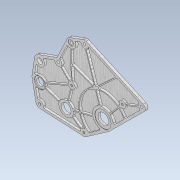
# Autodesk Inventor part: 脚フレーム内側後改
Saved by Autodesk Inventor 2020.2 (Build 242310000, 310)
## iProperties
Created: 2020-02-04
Part Number: 脚フレーム内側後改
Material: アルミニウム 7075
Document SubType Name: Modeling
Designer: aoyam
Density: 2.81 g/cm^3
Appearance: サテン - ブラシ仕上げ 重厚
Mass: 23.6517 g
Surface Area: 186.096 cm^2
Volume: 8.41698 cm^3
Author: aoyam
Autodesk Inventor part; units mm, degrees
ref_plane "YZ Plane" through (0, 0, 0) normal (1, 0, 0) x (0, 1, 0)
ref_plane "XZ Plane" through (0, 0, 0) normal (0, 1, 0) x (-1, 0, 0)
ref_plane "XY Plane" through (0, 0, 0) normal (0, 0, 1) x (1, 0, 0)
sketch "スケッチ2" plane through (0, 0, 0) normal (0, 0, 1) x (1, 0, 0)
  line L0 (0, 0) -> (0, 13.1)
  line L1 (26.2, 7.30753) -> (26.2, 0)
  line L2 (-139.706094, -70) -> (112.711025, -70)
  line L3 (-139.706094, -20) -> (112.711025, -20)
  line L4 (-139.723118, -25) -> (112.694001, -25)
  circle A0 centre (0, 0) radius 20.05
  circle A1 centre (14.844729, 16.628971) radius 2.05
  circle A2 centre (14.844729, 16.628971) radius 14
  circle A3 centre (19.387849, -11) radius 2.05
  circle A4 centre (19.387849, -11) radius 14
  circle A5 centre (0, 0) radius 9.1
  line L5 (0, 0) -> (-93.6, 0)
  circle A6 centre (-93.6, 0) radius 25.1
  circle A7 centre (-52.665625, 10.257531) radius 17.1
  circle A8 centre (-23.2, 0) radius 14.1
  line L6 (0, 0) -> (93.6, 0)
  circle A9 centre (93.6, 0) radius 25.1
  circle A10 centre (52.665625, 10.257531) radius 17.1
  circle A11 centre (23.2, 0) radius 14.1
  dimension "d137" = 7.30753
  dimension "d142" = 70
  dimension "d143" = 50
  dimension "d145" = 45
  dimension "d153" = 4.1
  dimension "d154" = 28
  dimension "d155" = 4.1
  dimension "d156" = 28
  dimension "d157" = 22.291
  dimension "d158" = 22.291
  dimension "d159" = 40.1
  dimension "d160" = 18.2
  dimension "d161" = 93.6
  dimension "d162" = 50.2
  dimension "d164" = 34.2
  dimension "d165" = 28.2
  constraints: 14 end point, 12 centre point, 7 coincident, 5 tangent, 4 symmetric about line, 2 horizontal, 2 parallel, 2 point on line, 1 vertical, 3 other
  measures "d137" distance of L1.start L1.end
  measures "d142" distance from line of L2 point (0, 0)
  measures "d143" distance between parallel lines of L2 L3
  measures "d145" distance between parallel lines of L2 L4
  measures "d153" diameter of A1
  measures "d154" diameter of A2
  measures "d155" diameter of A3
  measures "d156" diameter of A4
  measures "d157" distance of A1.centre point (0, 0)
  measures "d158" distance of A3.centre point (0, 0)
  measures "d159" diameter of A0
  measures "d160" diameter of A5
  measures "d161" distance of L0.start L5.end
  measures "d162" diameter of A6
  measures "d164" diameter of A7
  measures "d165" diameter of A8
sketch "スケッチ6" plane through (0, 0, 0) normal (0, 0, 1) x (1, 0, 0)
  circle A0 centre (93.6, 0) radius 6.025
  circle A1 centre (93.788626, 0) radius 8.025
  circle A2 centre (23.2, 0) radius 4
  circle A3 centre (23.2, 0) radius 14.1 construction
  circle A4 centre (93.6, 0) radius 25.1 construction
  circle A5 centre (23.2, 0) radius 16 construction
  circle A6 centre (93.6, 0) radius 27 construction
  line L0 (93.6, 0) -> (43.961305, 30) construction
  line L1 (43.961305, 30) -> (43.961305, 0) construction
  line L2 (93.6, 0) -> (0, 0)
  circle A7 centre (43.961305, 30) radius 1.5
  circle A8 centre (52.665625, -10.257531) radius 5.5
  circle A9 centre (52.665625, -10.257531) radius 17.1 construction
  circle A10 centre (52.665625, -10.257531) radius 19 construction
  line L3 (10.458367, 21.878509) -> (52.665625, 69.111596)
  line L4 (10.458367, -13.121491) -> (10.458367, 21.878509)
  line L5 (25.458367, -28.121491) -> (10.458367, -13.121491)
  line L6 (95.208425, -28.121491) -> (25.458367, -28.121491)
  line L7 (52.665625, 69.111596) -> (73.258556, 65.895552)
  line L8 (73.258556, 65.895552) -> (144.272455, 39.050636)
  line L9 (144.272455, 39.050636) -> (95.208425, -28.121491)
  circle A11 centre (73.258556, 61.870258) radius 1.5
  circle A12 centre (136.685646, 33.221118) radius 1.5
  line L10 (24.034996, -23.055024) -> (45.351309, -15.50165)
  arc A13 (45.351309, -15.50165) -> (58.061671, -17.460495) centre (52.665625, -10.257531) ccw
  line L11 (58.061671, -17.460495) -> (71.015612, -25.49562)
  arc A14 (71.015612, -25.49562) -> (74.255733, -25.093314) centre (72.402373, -23.4155) ccw
  line L12 (74.255733, -25.093314) -> (88.955218, -8.855845)
  arc A15 (88.955218, -8.855845) -> (101.830891, 5.679122) centre (93.6, 0) ccw
  line L13 (101.830891, 5.679122) -> (117.034634, 23.219838)
  arc A16 (117.034634, 23.219838) -> (113.256379, 26.49471) centre (115.145507, 24.857274) ccw
  line L14 (113.256379, 26.49471) -> (98.052637, 8.953995)
  arc A17 (98.052637, 8.953995) -> (85.704965, 6.13746) centre (93.6, 0) ccw
  line L15 (85.704965, 6.13746) -> (59.901593, 17.294675)
  arc A18 (59.901593, 17.294675) -> (59.314048, 17.467033) centre (58.90939, 15) ccw
  line L16 (59.314048, 17.467033) -> (23.604658, 23.324307)
  arc A19 (23.604658, 23.324307) -> (20.7, 20.857274) centre (23.2, 20.857274) ccw
  line L17 (20.7, 20.857274) -> (20.7, 5.454356)
  arc A20 (20.7, 5.454356) -> (20.7, -5.454356) centre (23.2, 0) ccw
  line L18 (20.7, -5.454356) -> (20.7, -20.69859)
  arc A21 (20.7, -20.69859) -> (24.034996, -23.055024) centre (23.2, -20.69859) ccw
  line L19 (25.7, 5.454356) -> (25.7, 17.913801)
  line L20 (25.7, 17.913801) -> (55.832623, 12.971263)
  line L21 (55.832623, 12.971263) -> (51.789591, -1.300268)
  arc A22 (51.789591, -1.300268) -> (43.681318, -10.788782) centre (52.665625, -10.257531) ccw
  line L22 (43.681318, -10.788782) -> (25.7, -17.16041)
  line L23 (25.7, -17.16041) -> (25.7, -5.454356)
  arc A23 (25.7, -5.454356) -> (25.7, 5.454356) centre (23.2, 0) ccw
  circle A24 centre (58.90939, 15) radius 1.5
  circle A25 centre (72.402373, -23.4155) radius 1.5
  circle A26 centre (23.2, 20.857274) radius 3
  circle A27 centre (115.145507, 24.857274) radius 1.5
  circle A28 centre (23.2, -20.69859) radius 1.5
  circle A29 centre (23.2, 0) radius 5
  circle A30 centre (93.6, 0) radius 5.525 construction
  line L24 (57.614258, -2.740149) -> (61.452441, 12.786227)
  line L25 (61.452441, 12.786227) -> (84.545331, 2.801007)
  arc A31 (84.545331, 2.801007) -> (85.779798, -5.785259) centre (94.081299, -0.209859) ccw
  line L26 (85.779798, -5.785259) -> (73.014253, -20.85157)
  line L27 (73.014253, -20.85157) -> (61.080634, -13.449335)
  arc A32 (61.080634, -13.449335) -> (57.614258, -2.740149) centre (52.665625, -10.257531) ccw
  circle A33 centre (52.665625, -10.257531) radius 4
  line L28 (6.354093, -32.225765) -> (150, -32.225765)
  line L29 (150, -32.225765) -> (150, 70)
  line L30 (150, 70) -> (6.354093, 70)
  line L31 (6.354093, 70) -> (6.354093, -32.225765)
  point P0 (52.665625, 10.257531)
  dimension "d166" = 12.05
  dimension "d167" = 16.05
  dimension "d169" = 8
  dimension "d170" = 28.2
  dimension "d172" = 50.2
  dimension "d173" = 32
  dimension "d175" = 54
  dimension "d176" = 58
  dimension "d177" = 30
  dimension "d178" = 3
  dimension "d191" = 34.2
  dimension "d220" = 6
  dimension "d456" = 2.5
  dimension "d457" = 3
  dimension "d458" = 2.5
  dimension "d459" = 3
  dimension "d460" = 3
  dimension "d461" = 2.5
  dimension "d462" = 2.5
  dimension "d463" = 1
  dimension "d464" = 5
  dimension "d465" = 5
  dimension "d466" = 5
  dimension "d467" = 5
  dimension "d468" = 11
  dimension "d469" = 3.5
  dimension "d470" = 3.5
  dimension "d471" = 3.5
  dimension "d472" = 2
  dimension "d473" = 2
  constraints: 64 end point, 32 centre point, 26 point on circle, 13 concentric, 5 coincident, 3 horizontal, 3 vertical, 2 parallel, 2 tangent, 1 perpendicular, 1 point on line, 5 other
  measures "d166" diameter of A0
  measures "d167" diameter of A1
  measures "d169" diameter of A2
  measures "d170" diameter of A3
  measures "d172" diameter of A4
  measures "d173" diameter of A5
  measures "d175" diameter of A6
  measures "d176" distance of L0.start L0.end
  measures "d177" distance of L0.end L1.end
  measures "d178" diameter of A7
  measures "d191" diameter of A9
  measures "d220" diameter of A26
  measures "d456" radius of A19
  measures "d457" diameter of A28
  measures "d458" radius of A21
  measures "d459" diameter of A24
  measures "d460" diameter of A25
  measures "d461" radius of A14
  measures "d462" radius of A16
  measures "d463" radial gap between concentric circles of A27 A16
  measures "d464" distance between parallel lines of L19 L17
  measures "d465" distance between parallel lines of L23 L18
  measures "d466" distance between parallel lines of L10 L22
  measures "d467" distance between parallel lines of L27 L11
  measures "d468" diameter of A8
  measures "d469" radial gap between concentric circles of A8 A22
  measures "d470" radial gap between concentric circles of A32 A8
  measures "d471" radial gap between concentric circles of A13 A8
  measures "d472" radial gap between concentric circles of A2 A20
  measures "d473" radial gap between concentric circles of A23 A2
extrude "押し出し4" add sketch "スケッチ6" along normal blind 3 contours A1 | L2 A29 A2 | A2 L2 A29 | A31 L26 L27 A32 L24 L2 | L2 L24 L25 A31 | L21 A22 L22 L23 A23 L2 | L2 A23 L19 L20 L21 | L3 L7 L8 L9 L6 L5 L4 | A21 L18 A20 L17 A26 L16 A18 L15 A17 L14 A16 L13 A15 L12 A14 L11 A13 L10 | A26 L16 A19 L17 | L17 A19 L16 A26 | A24 | A25 | A27 | A28 | L31 L30 L29 L28
sketch "スケッチ7" plane through (0, 0, 3) normal (0, 0, 1) x (1, 0, 0)
  circle A0 centre (52.665625, -10.257531) radius 5.5
  circle A1 centre (23.2, 0) radius 4
  circle A2 centre (52.665625, -10.257531) radius 6.1
  circle A3 centre (23.2, 0) radius 6
  point P0 (0, 0)
  point P1 (93.788626, 0)
  dimension "d184" = 0.6
  dimension "d481" = 12
  constraints: 2 centre point, 1 coincident
  measures "d184" radial gap between concentric circles of A0 A2
  measures "d481" diameter of A3
sketch "スケッチ8" plane through (0, 0, 3) normal (0, 0, 1) x (1, 0, 0)
  circle A0 centre (93.6, 0) radius 6.025 projected
  circle A1 centre (93.6, 0) radius 9.025
  point P0 (0, 0)
  dimension "d187" = 12.05
  dimension "d188" = 18.05
  constraints: 1 centre point, 1 coincident
  measures "d187" diameter of A0
  measures "d188" diameter of A1
extrude "押し出し6" cut sketch "スケッチ8" against normal blind 0.5
sketch "スケッチ9" plane through (0, 0, 3) normal (0, 0, 1) x (1, 0, 0)
  line L0 (24.034996, -23.055024) -> (46.835618, -14.97569)
  arc A0 (46.835618, -14.97569) -> (57.16233, -16.260001) centre (52.665625, -10.257531) ccw
  line L1 (57.16233, -16.260001) -> (71.015612, -25.49562)
  arc A1 (71.015612, -25.49562) -> (74.255733, -25.093314) centre (72.402373, -23.4155) ccw
  line L2 (74.255733, -25.093314) -> (88.955218, -8.855845)
  arc A2 (88.955218, -8.855845) -> (101.830891, 5.679122) centre (93.6, 0) ccw
  line L3 (101.830891, 5.679122) -> (117.034634, 23.219838)
  arc A3 (117.034634, 23.219838) -> (113.256379, 26.49471) centre (115.145507, 24.857274) ccw
  line L4 (113.256379, 26.49471) -> (98.052637, 8.953995)
  arc A4 (98.052637, 8.953995) -> (85.704965, 6.13746) centre (93.6, 0) ccw
  line L5 (85.704965, 6.13746) -> (59.901593, 17.294675)
  arc A5 (59.901593, 17.294675) -> (59.314048, 17.467033) centre (58.90939, 15) ccw
  line L6 (59.314048, 17.467033) -> (23.604658, 23.324307)
  arc A6 (23.604658, 23.324307) -> (20.7, 20.857274) centre (23.2, 20.857274) ccw
  line L7 (20.7, 20.857274) -> (20.7, 7.599342)
  arc A7 (20.7, 7.599342) -> (20.7, -7.599342) centre (23.2, 0) ccw
  line L8 (20.7, -7.599342) -> (20.7, -20.69859)
  arc A8 (20.7, -20.69859) -> (24.034996, -23.055024) centre (23.2, -20.69859) ccw
  line L9 (25.7, 7.599342) -> (25.7, 17.913801)
  line L10 (25.7, 17.913801) -> (55.832623, 12.971263)
  line L11 (55.832623, 12.971263) -> (51.935597, -2.793145)
  arc A9 (51.935597, -2.793145) -> (45.165627, -10.262821) centre (52.665625, -10.257531) ccw
  line L12 (45.165627, -10.262821) -> (25.7, -17.16041)
  line L13 (25.7, -17.16041) -> (25.7, -7.599342)
  arc A10 (25.7, -7.599342) -> (25.7, 7.599342) centre (23.2, 0) ccw
  circle A11 centre (58.90939, 15) radius 1.5
  circle A12 centre (72.402373, -23.4155) radius 1.5
  circle A13 centre (23.2, 20.857274) radius 1.5
  circle A14 centre (115.145507, 24.857274) radius 1.5
  circle A15 centre (23.2, -20.69859) radius 1.5
  circle A16 centre (23.150308, 0) radius 5
  circle A17 centre (93.6, 0) radius 5.525
  line L14 (56.789486, -3.993046) -> (60.627669, 11.53333)
  line L15 (60.627669, 11.53333) -> (83.720559, 1.54811)
  arc A18 (83.720559, 1.54811) -> (85.248498, -5.500219) centre (93.6, 0) ccw
  line L16 (85.248498, -5.500219) -> (71.995637, -20.139705)
  line L17 (71.995637, -20.139705) -> (59.935851, -12.099763)
  arc A19 (59.935851, -12.099763) -> (56.789486, -3.993046) centre (52.665625, -10.257531) ccw
  circle A20 centre (52.665625, -10.257531) radius 4
  circle A21 centre (23.2, 20.857274) radius 3
  circle A22 centre (58.90939, 15) radius 1.25
  circle A23 centre (23.2, -20.69859) radius 1.5
  circle A24 centre (72.402373, -23.4155) radius 1.25
  circle A25 centre (115.145507, 24.857274) radius 1.25
  point P0 (0, 0)
  point P1 (0, 0)
  dimension "d192" = 6
  dimension "d194" = 2.5
  dimension "d195" = 3
  dimension "d196" = 2.5
  dimension "d197" = 2.5
  constraints: 36 end point, 26 centre point, 26 point on circle, 5 coincident, 4 vertical, 89 other
  measures "d192" diameter of A21
  measures "d194" diameter of A22
  measures "d195" diameter of A23
  measures "d196" diameter of A24
  measures "d197" diameter of A25
extrude "押し出し7" cut sketch "スケッチ9" against normal blind 3 contours A21 L6 A6 L7 | L7 A6 L6 A21 | A13 | A15 | A22 | A24 | A25
thread "ねじ1" size "M3x0.5" class "6H" standard "ANSI Metric M Profile" full length
thread "ねじ2" size "M3x0.5" class "6H" standard "ANSI Metric M Profile" full length
thread "ねじ3" size "M3x0.5" class "6H" standard "ANSI Metric M Profile" full length
sketch "スケッチ12" plane through (0, 0, 3) normal (0, 0, 1) x (1, 0, 0)
  circle A0 centre (136.685646, 33.221118) radius 1.5
  circle A1 centre (73.258556, 61.870258) radius 1.5
  circle A2 centre (43.961305, 30) radius 1.5
  circle A3 centre (93.6, 0) radius 9.025
  circle A4 centre (23.2, 20.857274) radius 3
  circle A5 centre (115.145507, 24.857274) radius 1.25
  circle A6 centre (23.2, -20.69859) radius 1.5
  circle A7 centre (72.402373, -23.4155) radius 1.25
  circle A8 centre (58.90939, 15) radius 1.25
  point P0 (0, 0)
sketch "後ろダンパー" plane through (0, 0, 3) normal (0, 0, 1) x (1, 0, 0)
  circle A0 centre (27.117906, 46.680777) radius 5.0025
  circle A1 centre (17.304254, 39.743183) radius 1.5
  line L0 (17.304254, 39.743183) -> (-58.013111, 55.752383)
  circle A2 centre (-58.013111, 55.752383) radius 1.25
  line L1 (0, 0) -> (0, 16.677732)
  circle A3 centre (58.013111, 55.752383) radius 1.25
  circle A4 centre (58.013111, 55.752383) radius 1.5
  circle A5 centre (23.2, 0) radius 5
  line L2 (58.013111, 55.752383) -> (23.2, 0)
  line L3 (42.438218, 62.997595) -> (23.2, 0)
  line L4 (23.2, 0) -> (72.547914, 46.047257)
  circle A6 centre (42.438218, 62.997595) radius 62
  circle A7 centre (42.438218, 62.997595) radius 91
  circle A8 centre (72.547914, 46.047257) radius 91
  circle A9 centre (72.547914, 46.047257) radius 62
  dimension "d273" = 77
  dimension "d275" = 2.5
  dimension "d377" = 3
  dimension "d378" = 15
  dimension "d379" = 15
  dimension "d380" = 124
  dimension "d381" = 182
  dimension "d382" = 182
  dimension "d383" = 124
  constraints: 10 end point, 9 centre point, 6 coincident, 1 symmetric about line, 1 vertical, 4 other
  measures "d273" distance of L0.start L0.end
  measures "d275" diameter of A2
  measures "d377" diameter of A4
  measures "d378" angle of L2 L3
  measures "d379" angle of L4 L2
  measures "d380" diameter of A6
  measures "d381" diameter of A7
  measures "d382" diameter of A8
  measures "d383" diameter of A9
extrude "押し出し11" cut sketch "後ろダンパー" against normal blind 10 contours A3 | A4
sketch "スケッチ15" plane through (0, 0, 3) normal (0, 0, 1) x (1, 0, 0)
  circle A0 centre (58.013111, 55.752383) radius 3
  circle A1 centre (58.013111, 55.752383) radius 1.5
  point P0 (0, 0)
  point P1 (43.961305, 30)
  point P2 (47.596697, 40.144096)
  point P3 (56.056816, 55.33656)
  dimension "d276" = 6
  constraints: 1 centre point, 1 coincident, 1 concentric
  measures "d276" diameter of A0
extrude "押し出し12" cut sketch "スケッチ15" against normal blind 0.5 contours A0 | A1
sketch "スケッチ16" plane through (0, 0, 3) normal (0, 0, 1) x (1, 0, 0)
  circle A0 centre (23.2, 20.857274) radius 3
  point P0 (0, 0)
sketch "スケッチ17" plane through (0, 0, 3) normal (0, 0, 1) x (1, 0, 0)
  circle A0 centre (58.013111, 55.752383) radius 4.5
  circle A1 centre (58.90939, 15) radius 1.25
  circle A2 centre (72.402373, -23.4155) radius 1.25
  circle A3 centre (23.2, -20.69859) radius 1.5
  circle A4 centre (115.145507, 24.857274) radius 1.25
  circle A5 centre (23.2, 20.857274) radius 3
  circle A6 centre (93.6, 0) radius 9.025
  circle A7 centre (43.961305, 30) radius 1.5
  circle A8 centre (73.258556, 61.870258) radius 1.5
  circle A9 centre (136.685646, 33.221118) radius 1.5
  line L0 (6.354093, -32.225765) -> (150, -32.225765)
  line L1 (150, -32.225765) -> (150, 70)
  line L2 (150, 70) -> (6.354093, 70)
  line L3 (6.354093, 70) -> (6.354093, -32.225765)
  circle A10 centre (23.2, 20.857274) radius 5.5
  circle A11 centre (23.040638, 1.791605) radius 8.298679
  circle A12 centre (23.2, -20.69859) radius 4
  circle A13 centre (72.402373, -23.4155) radius 3.75
  circle A14 centre (93.6, 0) radius 10.775
  circle A15 centre (136.685646, 33.221118) radius 4
  circle A16 centre (73.258556, 61.870258) radius 4
  circle A17 centre (43.961305, 30) radius 4
  line L4 (21.321043, 26.026367) -> (42.594791, 33.75934)
  line L5 (42.594791, 33.75934) -> (53.947689, 57.68172)
  line L6 (56.465094, 59.97774) -> (71.882541, 65.626131)
  line L7 (74.905125, 65.515641) -> (138.332215, 36.866501)
  line L8 (139.503558, 30.382215) -> (101.19075, -7.647296)
  line L9 (99.77954, -8.826886) -> (74.553025, -26.487503)
  line L10 (72.214615, -27.160797) -> (22.999725, -24.693573)
  line L11 (19.279257, -21.490914) -> (14.906392, 0.147794)
  line L12 (17.766513, 21.710044) -> (14.842317, 3.078308)
  circle A18 centre (58.013111, 55.752383) radius 3
  line L13 (140.681024, 33.02888) -> (141.188535, 43.576709) construction
  line L14 (74.420443, 65.697792) -> (139.411825, 45.968987) construction
  line L15 (122.455421, 48.634428) -> (138.685646, 43.576779) construction
  line L16 (122.009158, 47.202349) -> (138.239383, 42.1447) construction
  line L17 (139.131909, 45.008857) -> (122.901685, 50.066507) construction
  circle A19 centre (122.455421, 48.634428) radius 1.5 construction
  circle A20 centre (138.685646, 43.576779) radius 1.5 construction
  circle A21 centre (138.685646, 43.576779) radius 2.5 construction
  circle A22 centre (93.6, 0) radius 6.025
  circle A23 centre (23.2, 0) radius 4
  point P0 (0, 0)
  point P1 (41.137344, 33.229561)
  point P2 (71.208303, 65.876062)
  point P3 (104.018487, -6.004644)
  point P4 (74.869918, -26.875808)
  point P5 (55.236344, 56.963455)
  point P6 (57.020921, 58.61467)
  point P7 (72.510099, 65.799611)
  point P8 (74.597345, 66.166494)
  point P9 (130.570534, 46.105603)
  point P10 (141.182757, 43.45663)
  dimension "d374" = 5
  dimension "d277" = 2.5
  dimension "d279" = 2.5
  dimension "d280" = 2.5
  dimension "d282" = 1.75
  dimension "d283" = 2.5
  dimension "d284" = 2.5
  dimension "d286" = 2.5
  dimension "d371" = 7.42183
  dimension "d372" = 17
  dimension "d373" = 3
  dimension "d390" = 1.5
  dimension "d423" = 17.308
  dimension "d474" = 2.5
  constraints: 30 end point, 23 point on circle, 22 tangent, 19 centre point, 1 coincident, 1 concentric, 1 midpoint, 1 parallel, 10 other
  measures "d277" radial gap between concentric circles of A8 A16
  measures "d280" radial gap between concentric circles of A9 A15
  measures "d282" radial gap between concentric circles of A14 A6
  measures "d283" radial gap between concentric circles of A13 A2
  measures "d284" radial gap between concentric circles of A12 A3
  measures "d286" radial gap between concentric circles of A5 A10
  measures "d371" angle of L7 L14
  measures "d372" distance of L15.start L15.end
  measures "d373" diameter of A20
  measures "d390" radial gap between concentric circles of A0 A18
  measures "d423" angle of L15 L2
sketch "スケッチ17 outline for 押し出し16" plane through (0, 0, 3) normal (0, 0, 1) x (1, 0, 0)
  line L0 (6.354093, -32.225765) -> (150, -32.225765)
  line L1 (6.354093, 70) -> (6.354093, -32.225765)
  line L2 (150, -32.225765) -> (150, 70)
  line L3 (150, 70) -> (6.354093, 70)
  line L4 (14.842317, 3.078308) -> (17.766513, 21.710044)
  arc A0 (14.906392, 0.147794) -> (14.842317, 3.078308) centre (23.040638, 1.791605) cw
  line L5 (19.279257, -21.490914) -> (14.906392, 0.147794)
  arc A1 (22.999725, -24.693573) -> (19.279257, -21.490914) centre (23.2, -20.69859) cw
  line L6 (72.214615, -27.160797) -> (22.999725, -24.693573)
  arc A2 (74.553025, -26.487503) -> (72.214615, -27.160797) centre (72.402373, -23.4155) cw
  line L7 (99.77954, -8.826886) -> (74.553025, -26.487503)
  arc A3 (101.19075, -7.647296) -> (99.77954, -8.826886) centre (93.6, 0) cw
  line L8 (139.503558, 30.382215) -> (101.19075, -7.647296)
  arc A4 (138.332215, 36.866501) -> (139.503558, 30.382215) centre (136.685646, 33.221118) cw
  line L9 (74.905125, 65.515641) -> (138.332215, 36.866501)
  arc A5 (71.882541, 65.626131) -> (74.905125, 65.515641) centre (73.258556, 61.870258) cw
  line L10 (56.465094, 59.97774) -> (71.882541, 65.626131)
  arc A6 (53.947689, 57.68172) -> (56.465094, 59.97774) centre (58.013111, 55.752383) cw
  line L11 (42.594791, 33.75934) -> (53.947689, 57.68172)
  line L12 (21.321043, 26.026367) -> (42.594791, 33.75934)
  arc A7 (17.766513, 21.710044) -> (21.321043, 26.026367) centre (23.2, 20.857274) cw
extrude "押し出し16" cut sketch "スケッチ17 outline for 押し出し16" against normal blind 10
sketch "スケッチ18" plane through (0, 0, 3) normal (0, 0, 1) x (1, 0, 0)
  line L0 (14.906392, 0.147794) -> (19.279257, -21.490914)
  arc A0 (19.279257, -21.490914) -> (22.999725, -24.693573) centre (23.2, -20.69859) ccw
  line L1 (22.999725, -24.693573) -> (72.214615, -27.160797)
  arc A1 (72.214615, -27.160797) -> (74.553025, -26.487503) centre (72.402373, -23.4155) ccw
  line L2 (74.553025, -26.487503) -> (99.77954, -8.826886)
  arc A2 (99.77954, -8.826886) -> (101.19075, -7.647296) centre (93.6, 0) ccw
  line L3 (101.19075, -7.647296) -> (139.503558, 30.382215)
  arc A3 (139.503558, 30.382215) -> (138.332215, 36.866501) centre (136.685646, 33.221118) ccw
  line L4 (138.332215, 36.866501) -> (74.905125, 65.515641)
  arc A4 (74.905125, 65.515641) -> (71.882541, 65.626131) centre (73.258556, 61.870258) ccw
  line L5 (71.882541, 65.626131) -> (56.465094, 59.97774)
  arc A5 (56.465094, 59.97774) -> (53.947689, 57.68172) centre (58.013111, 55.752383) ccw
  line L6 (53.947689, 57.68172) -> (42.594791, 33.75934)
  line L7 (42.594791, 33.75934) -> (21.321043, 26.026367)
  arc A6 (21.321043, 26.026367) -> (17.766513, 21.710044) centre (23.2, 20.857274) ccw
  line L8 (17.766513, 21.710044) -> (14.842317, 3.078308)
  arc A7 (14.842317, 3.078308) -> (14.906392, 0.147794) centre (23.040638, 1.791605) ccw
  circle A8 centre (58.013111, 55.752383) radius 3
  circle A9 centre (58.90939, 15) radius 1.25
  circle A10 centre (72.402373, -23.4155) radius 1.25
  circle A11 centre (23.2, -20.69859) radius 1.5
  circle A12 centre (115.145507, 24.857274) radius 1.25
  circle A13 centre (23.2, 20.857274) radius 3
  circle A14 centre (93.6, 0) radius 9.025
  circle A15 centre (43.961305, 30) radius 1.5
  circle A16 centre (73.258556, 61.870258) radius 1.5
  circle A17 centre (136.685646, 33.221118) radius 1.5
  line L9 (73.876019, 63.237277) -> (137.303109, 34.588137)
  arc A18 (137.742363, 32.15653) -> (137.303109, 34.588137) centre (136.685646, 33.221118) ccw
  line L10 (137.742363, 32.15653) -> (99.429555, -5.872982)
  arc A19 (98.345772, -6.778885) -> (99.429555, -5.872982) centre (93.6, 0) ccw
  line L11 (98.345772, -6.778885) -> (73.119257, -24.439501)
  arc A20 (72.339787, -24.663933) -> (73.119257, -24.439501) centre (72.402373, -23.4155) ccw
  line L12 (72.339787, -24.663933) -> (23.124897, -22.196709)
  arc A21 (21.729722, -20.995712) -> (23.124897, -22.196709) centre (23.2, -20.69859) ccw
  line L13 (21.729722, -20.995712) -> (17.356856, 0.642996)
  arc A22 (17.312084, 2.690685) -> (17.356856, 0.642996) centre (23.040638, 1.791605) ccw
  line L14 (17.312084, 2.690685) -> (20.23628, 21.322421)
  arc A23 (22.175114, 23.676779) -> (20.23628, 21.322421) centre (23.2, 20.857274) ccw
  line L15 (22.175114, 23.676779) -> (44.413365, 31.760348)
  line L16 (44.413365, 31.760348) -> (56.206257, 56.609866)
  arc A24 (57.325103, 57.63032) -> (56.206257, 56.609866) centre (58.013111, 55.752383) ccw
  line L17 (57.325103, 57.63032) -> (72.74255, 63.278711)
  arc A25 (73.876019, 63.237277) -> (72.74255, 63.278711) centre (73.258556, 61.870258) ccw
  circle A26 centre (23.2, 0) radius 6.5
  circle A27 centre (23.2, 20.857274) radius 5.5
  circle A28 centre (93.6, 0) radius 11.525
  circle A29 centre (58.90939, 15) radius 3.75
  circle A30 centre (43.961305, 30) radius 4
  circle A31 centre (58.013111, 55.752383) radius 5.5
  circle A32 centre (73.258556, 61.870258) radius 4
  circle A33 centre (115.145507, 24.857274) radius 3.75
  circle A34 centre (136.685646, 33.221118) radius 4
  circle A35 centre (52.665625, -10.257531) radius 8
  circle A36 centre (23.2, -20.69859) radius 4
  circle A37 centre (72.402373, -23.4155) radius 3.75
  circle A38 centre (93.6, 0) radius 27
  circle A39 centre (93.6, 0) radius 26
  line L18 (43.961305, 30) -> (58.90939, 15) construction
  line L19 (43.60714, 29.64706) -> (58.555224, 14.64706)
  line L20 (59.263555, 15.35294) -> (44.315471, 30.35294)
  arc A40 (44.315471, 30.35294) -> (43.60714, 29.64706) centre (43.961305, 30) ccw
  arc A41 (58.555224, 14.64706) -> (59.263555, 15.35294) centre (58.90939, 15) ccw
  line L21 (58.90939, 15) -> (52.665625, -10.257531) construction
  line L22 (58.424001, 15.11999) -> (52.180236, -10.137541)
  line L23 (53.151014, -10.377521) -> (59.394779, 14.88001)
  arc A42 (59.394779, 14.88001) -> (58.424001, 15.11999) centre (58.90939, 15) ccw
  arc A43 (52.180236, -10.137541) -> (53.151014, -10.377521) centre (52.665625, -10.257531) ccw
  line L24 (52.665625, -10.257531) -> (23.2, 0) construction
  line L25 (52.830009, -9.785326) -> (23.364384, 0.472206)
  line L26 (23.035616, -0.472206) -> (52.501241, -10.729737)
  arc A44 (52.501241, -10.729737) -> (52.830009, -9.785326) centre (52.665625, -10.257531) ccw
  arc A45 (23.364384, 0.472206) -> (23.035616, -0.472206) centre (23.2, 0) ccw
  line L27 (72.402373, -23.4155) -> (52.665625, -10.257531) construction
  line L28 (72.679725, -22.999477) -> (52.942977, -9.841507)
  line L29 (52.388273, -10.673555) -> (72.125021, -23.831524)
  arc A46 (72.125021, -23.831524) -> (72.679725, -22.999477) centre (72.402373, -23.4155) ccw
  arc A47 (52.942977, -9.841507) -> (52.388273, -10.673555) centre (52.665625, -10.257531) ccw
  line L30 (93.6, 0) -> (52.665625, -10.257531) construction
  line L31 (93.478465, 0.485004) -> (52.54409, -9.772527)
  line L32 (52.78716, -10.742535) -> (93.721535, -0.485004)
  arc A48 (93.721535, -0.485004) -> (93.478465, 0.485004) centre (93.6, 0) ccw
  arc A49 (52.54409, -9.772527) -> (52.78716, -10.742535) centre (52.665625, -10.257531) ccw
  line L33 (58.013111, 55.752383) -> (58.90939, 15) construction
  line L34 (57.513232, 55.741389) -> (58.409511, 14.989006)
  line L35 (59.409269, 15.010994) -> (58.51299, 55.763377)
  arc A50 (58.51299, 55.763377) -> (57.513232, 55.741389) centre (58.013111, 55.752383) ccw
  arc A51 (58.409511, 14.989006) -> (59.409269, 15.010994) centre (58.90939, 15) ccw
  line L36 (73.258556, 61.870258) -> (93.6, 0) construction
  line L37 (72.783569, 61.714094) -> (93.125013, -0.156164)
  line L38 (94.074987, 0.156164) -> (73.733543, 62.026423)
  arc A52 (73.733543, 62.026423) -> (72.783569, 61.714094) centre (73.258556, 61.870258) ccw
  arc A53 (93.125013, -0.156164) -> (94.074987, 0.156164) centre (93.6, 0) ccw
  line L39 (93.6, 0) -> (115.145507, 24.857274) construction
  line L40 (93.977825, -0.327487) -> (115.523332, 24.529787)
  line L41 (114.767681, 25.184761) -> (93.222175, 0.327487)
  arc A54 (93.222175, 0.327487) -> (93.977825, -0.327487) centre (93.6, 0) ccw
  arc A55 (115.523332, 24.529787) -> (114.767681, 25.184761) centre (115.145507, 24.857274) ccw
  line L42 (115.145507, 24.857274) -> (136.685646, 33.221118) construction
  line L43 (115.326488, 24.391178) -> (136.866627, 32.755022)
  line L44 (136.504665, 33.687215) -> (114.964526, 25.32337)
  arc A56 (114.964526, 25.32337) -> (115.326488, 24.391178) centre (115.145507, 24.857274) ccw
  arc A57 (136.866627, 32.755022) -> (136.504665, 33.687215) centre (136.685646, 33.221118) ccw
  line L45 (58.46125, 35.376192) -> (85.16713, 25.649302) construction
  line L46 (58.290136, 34.906383) -> (84.996015, 25.179494)
  line L47 (85.338245, 26.11911) -> (58.632365, 35.846)
  arc A58 (58.632365, 35.846) -> (58.290136, 34.906383) centre (58.46125, 35.376192) ccw
  arc A59 (84.996015, 25.179494) -> (85.338245, 26.11911) centre (85.16713, 25.649302) ccw
  line L48 (85.16713, 25.649302) -> (108.50715, 47.594874) construction
  line L49 (85.509634, 25.285035) -> (108.849654, 47.230606)
  line L50 (108.164646, 47.959141) -> (84.824626, 26.01357)
  arc A60 (84.824626, 26.01357) -> (85.509634, 25.285035) centre (85.16713, 25.649302) ccw
  arc A61 (108.849654, 47.230606) -> (108.164646, 47.959141) centre (108.50715, 47.594874) ccw
  circle A62 centre (72.621951, -18.620525) radius 1.05
  line L51 (23.2, 0) -> (58.90939, 15) construction
  line L52 (23.393639, -0.460982) -> (59.103029, 14.539018)
  line L53 (58.715751, 15.460982) -> (23.006361, 0.460982)
  arc A63 (23.006361, 0.460982) -> (23.393639, -0.460982) centre (23.2, 0) ccw
  arc A64 (59.103029, 14.539018) -> (58.715751, 15.460982) centre (58.90939, 15) ccw
  circle A65 centre (23.2, 0) radius 4
  circle A66 centre (52.665625, -10.257531) radius 5.5
  point P0 (51.435348, 22.5)
  point P1 (55.787507, 2.371234)
  point P2 (37.932812, -5.128766)
  point P3 (62.533999, -16.836516)
  point P4 (73.132812, -5.128766)
  point P5 (83.429278, 30.935129)
  point P6 (104.372753, 12.428637)
  point P7 (125.915576, 29.039196)
  point P8 (71.81419, 30.512747)
  point P9 (96.83714, 36.622088)
  point P10 (84.416976, 25.390393)
  point P11 (58.977208, 34.656136)
  point P12 (59.32755, 18.726613)
  point P13 (58.502888, 11.272098)
  point P14 (55.067102, -2.626482)
  point P15 (60.28899, -7.831773)
  point P16 (67.292717, -6.076745)
  point P17 (73.407226, -17.9235)
  point P18 (67.535786, -7.046754)
  point P19 (60.53206, -8.801782)
  point P20 (59.586345, -14.270465)
  point P21 (69.587406, -20.937909)
  point P22 (72.573918, -19.669426)
  point P23 (82.552708, -3.283742)
  point P24 (68.505968, -6.803642)
  point P25 (78.154109, -20.914694)
  point P26 (91.774272, -11.37947)
  point P27 (111.004015, 19.315804)
  point P28 (101.5193, 8.37319)
  point P29 (105.122866, -0.221769)
  point P30 (116.922885, 11.490998)
  point P31 (89.528816, 10.78198)
  point P32 (85.005973, 24.538596)
  point P33 (68.262898, -5.833633)
  point P34 (82.309639, -2.313733)
  point P35 (100.763649, 9.028165)
  point P36 (110.248364, 19.970778)
  point P37 (85.955947, 24.850925)
  point P38 (90.47879, 11.094308)
  point P39 (133.167101, 31.318529)
  point P40 (118.790998, 25.736416)
  point P41 (113.089108, 21.721397)
  point P42 (111.659106, 20.071589)
  point P43 (117.669985, 12.232573)
  point P44 (135.110629, 29.544255)
  point P45 (108.962823, 47.389052)
  point P46 (86.248725, 25.979968)
  point P47 (110.903455, 20.726564)
  point P48 (112.333457, 22.376372)
  point P49 (118.429036, 26.668609)
  point P50 (132.805139, 32.250722)
  point P51 (133.923749, 36.114547)
  point P52 (85.396815, 26.551574)
  point P53 (108.014091, 47.817581)
  point P54 (77.255379, 61.710867)
  point P55 (74.973058, 58.25633)
  point P56 (58.953612, 35.728994)
  point P57 (84.370447, 26.471604)
  point P58 (74.023084, 57.944001)
  point P59 (69.260763, 62.003111)
  point P60 (62.135884, 59.392815)
  point P61 (58.633423, 50.287476)
  point P62 (57.633665, 50.265488)
  point P63 (54.00961, 51.981179)
  point P64 (45.356946, 33.748625)
  point P65 (47.116845, 27.541836)
  point P66 (56.640141, 17.985466)
  point P67 (58.327792, 18.704625)
  point P68 (29.484867, -1.658448)
  point P69 (45.289491, -7.160331)
  point P70 (54.096325, -2.386502)
  point P71 (57.53211, 11.512078)
  point P72 (55.931809, 17.279586)
  point P73 (46.408514, 26.835957)
  point P74 (39.963861, 30.14296)
  point P75 (26.50754, 25.251609)
  point P76 (19.521539, 16.768396)
  point P77 (17.326899, 2.785083)
  point P78 (69.032701, -21.769957)
  point P79 (59.03164, -15.102513)
  point P80 (44.960724, -8.104742)
  point P81 (29.1561, -2.602859)
  point P82 (18.364628, -4.343867)
  point P83 (20.995217, -17.361086)
  point P84 (26.828345, -22.382369)
  point P85 (68.808687, -24.486913)
  point P86 (41.054695, 7.5)
  point P87 (55.676537, 13.099695)
  point P88 (29.368643, 2.048864)
  point P89 (28.981365, 2.970827)
  point P90 (55.289259, 14.021658)
  dimension "d437" = 54
  dimension "d424" = 2.5
  dimension "d426" = 2.5
  dimension "d427" = 2.5
  dimension "d428" = 2.5
  dimension "d429" = 2.5
  dimension "d430" = 2.5
  dimension "d431" = 2.5
  dimension "d432" = 2.5
  dimension "d433" = 2.5
  dimension "d435" = 2.5
  dimension "d436" = 2.5
  dimension "d438" = 1
  dimension "d439" = 1
  dimension "d440" = 1
  dimension "d441" = 1
  dimension "d442" = 1
  dimension "d443" = 1
  dimension "d444" = 1
  dimension "d445" = 1
  dimension "d446" = 1
  dimension "d447" = 1
  dimension "d448" = 1
  dimension "d449" = 1
  dimension "d450" = 38
  dimension "d451" = 2.1
  dimension "d454" = 1
  dimension "d475" = 2.5
  dimension "d476" = 2.5
  constraints: 114 end point, 64 point on circle, 49 tangent, 46 centre point, 12 midpoint, 12 parallel, 2 point on line, 1 coincident, 20 other
  measures "d424" distance between parallel lines of L4 L9
  measures "d426" radial gap between concentric circles of A13 A27
  measures "d427" radial gap between concentric circles of A14 A28
  measures "d428" radial gap between concentric circles of A9 A29
  measures "d429" radial gap between concentric circles of A15 A30
  measures "d430" radial gap between concentric circles of A8 A31
  measures "d431" radial gap between concentric circles of A16 A32
  measures "d432" radial gap between concentric circles of A12 A33
  measures "d433" radial gap between concentric circles of A17 A34
  measures "d435" radial gap between concentric circles of A11 A36
  measures "d436" radial gap between concentric circles of A10 A37
  measures "d439" diameter of A41
  measures "d440" diameter of A43
  measures "d441" diameter of A45
  measures "d442" diameter of A47
  measures "d443" diameter of A49
  measures "d444" diameter of A51
  measures "d445" diameter of A53
  measures "d446" diameter of A55
  measures "d447" diameter of A57
  measures "d448" diameter of A59
  measures "d449" diameter of A61
  measures "d450" distance of L48.end L9.start
  measures "d451" diameter of A62
  measures "d454" diameter of A64
  measures "d475" radial gap between concentric circles of A65 A26
  measures "d476" radial gap between concentric circles of A66 A35
fillet "フィレット10" radius 1.05 1 edges at (42.5948, 33.7593, 1.5)
extrude "押し出し19" cut sketch "スケッチ18" against normal blind 2.5 contours L13 A26 L26 A35 L29 A37 L12 A36 | A27 L15 A30 L19 A29 L53 A26 L14 | A26 L52 A29 L22 A35 L25 | L16 A31 L34 A29 L20 A30 | L28 A35 L32 A38 A62 A37 | A39 L32 A28 L11 | A62 | L17 A32 L37 L47 L35 A31 | A38 L40 A33 L43 A34 L10 | L23 A29 L35 L46 A38 L31 A35 | A28 L40 A39 L10 | A39 L37 A28 L31 | A38 L49 A61 L9 A34 L44 A33 L41 | L9 L50 L38 A32 | A39 L41 A28 L38
fillet "フィレット11" radius 1.05 77 edges at (19.5215, 16.7684, 1.75) (26.5075, 25.2516, 1.75) (39.9639, 30.143, 1.75) (46.4085, 26.836, 1.75) (47.1168, 27.5418, 1.75) (45.3569, 33.7486, 1.75) (17.3269, 2.7851, 1.75) (28.9814, 2.9708, 1.75) (29.1561, -2.6029, 1.75) (29.4849, -1.6584, 1.75) (18.3646, -4.3439, 1.75) (20.9952, -17.3611, 1.75) (26.8283, -22.3824, 1.75) (59.0316, -15.1025, 1.75) (44.9607, -8.1047, 1.75) (45.2895, -7.1603, 1.75) (54.0963, -2.3865, 1.75) (55.0671, -2.6265, 1.75) (60.5321, -8.8018, 1.75) (60.289, -7.8318, 1.75) (59.5863, -14.2705, 1.75) (69.5874, -20.9379, 1.75) (69.0327, -21.77, 1.75) (68.8087, -24.4869, 1.75) (78.1541, -20.9147, 1.75) (68.506, -6.8036, 1.75) (67.5358, -7.0468, 1.75) (67.2927, -6.0767, 1.75) (68.2629, -5.8336, 1.75) (82.5527, -3.2837, 1.75) (82.3096, -2.3137, 1.75) (91.7743, -11.3795, 1.75) (105.1229, -0.2218, 1.75) (101.5193, 8.3732, 1.75) (100.7636, 9.0282, 1.75) (89.5288, 10.782, 1.75) (90.4788, 11.0943, 1.75) (84.3704, 26.4716, 1.75) (85.3968, 26.5516, 1.75) (85.006, 24.5386, 1.75) (84.417, 25.3904, 1.75) (85.9559, 24.8509, 1.75) (86.2487, 25.98, 1.75) (58.5029, 11.2721, 1.75) (57.5321, 11.5121, 1.75) (55.6765, 13.0997, 1.75) (55.2893, 14.0217, 1.75) (58.3278, 18.7046, 1.75) (59.3276, 18.7266, 1.75) (55.9318, 17.2796, 1.75) (56.6401, 17.9855, 1.75) (54.0096, 51.9812, 1.75) (57.6337, 50.2655, 1.75) (58.6334, 50.2875, 1.75) (62.1359, 59.3928, 1.75) (69.2608, 62.0031, 1.75) (74.0231, 57.944, 1.75) (74.9731, 58.2563, 1.75) (77.2554, 61.7109, 1.75) (108.9628, 47.3891, 1.75) (108.0141, 47.8176, 1.75) (133.9237, 36.1145, 1.75) (132.8051, 32.2507, 1.75) (133.1671, 31.3185, 1.75) (135.1106, 29.5443, 1.75) (116.9229, 11.491, 1.75) (117.67, 12.2326, 1.75) (113.0891, 21.7214, 1.75) (118.791, 25.7364, 1.75) (118.429, 26.6686, 1.75) (112.3335, 22.3764, 1.75) (110.9035, 20.7266, 1.75) (110.2484, 19.9708, 1.75) (111.6591, 20.0716, 1.75) (111.004, 19.3158, 1.75) (58.9536, 35.729, 1.75) (58.9772, 34.6561, 1.75)
sketch "ざぐり" plane through (0, 0, 0) normal (0, 0, -1) x (-1, 0, 0)
  circle A0 centre (-23.2, -20.69859) radius 1.5
  circle A1 centre (-23.2, -20.69859) radius 3
  point P0 (0, 0)
  dimension "d477" = 6
  constraints: 1 centre point, 1 coincident
  measures "d477" diameter of A1
chamfer "面取り1" distance 1.5 angle 45 1 edges at (21.7, -20.6986, 0)
extrude "押し出し20" cut sketch "スケッチ7" against normal blind 0.8 contours A3
